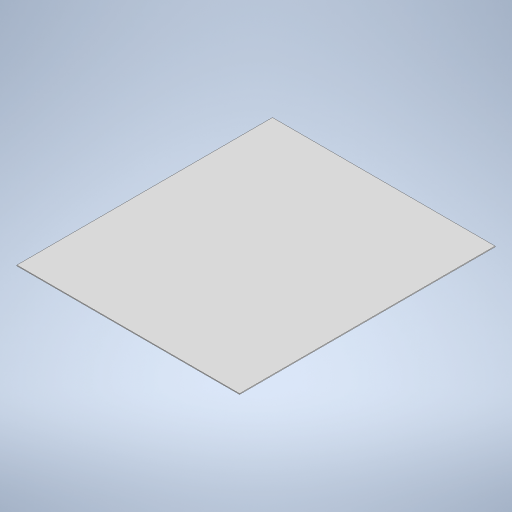
# Autodesk Inventor part: sheet
Saved by Autodesk Inventor 2023.1 (Build 271208000, 208)
## iProperties
Created: 2023-01-21
Part Number: sheet
Material: Generic
Document SubType Name: Modeling
Designer: eplym
Density: 1 g/cm^3
Appearance: Default
Author: eplym
Autodesk Inventor part; units mm, degrees
ref_plane "YZ Plane" through (0, 0, 0) normal (1, 0, 0) x (0, 1, 0)
ref_plane "XZ Plane" through (0, 0, 0) normal (0, 1, 0) x (-1, 0, 0)
ref_plane "XY Plane" through (0, 0, 0) normal (0, 0, 1) x (1, 0, 0)
sketch "Sketch1" plane through (0, 0, 0) normal (0, 1, 0) x (-1, 0, 0)
  line L0 (-220, 252.5) -> (220, 252.5)
  line L1 (220, 252.5) -> (220, -252.5)
  line L2 (220, -252.5) -> (-220, -252.5)
  line L3 (-220, -252.5) -> (-220, 252.5)
  line L4 (-220, 252.5) -> (220, -252.5) construction
  line L5 (220, 252.5) -> (-220, -252.5) construction
  point P0 (0, 0)
  dimension "d1" = 505
  dimension "d2" = 440
  constraints: 12 end point, 2 midpoint, 2 parallel, 1 horizontal, 1 perpendicular
  measures "d1" distance of L0.end L1.end
  measures "d2" distance of L1.end L2.end
extrude "Extrusion1" add sketch "Sketch1" along normal blind 1.6
body "Solid1"
